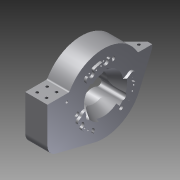
# Autodesk Inventor part: launcherhousing
Saved by Autodesk Inventor 2011 (Build 150239000, 239)
## iProperties
Created: 2011-01-27
Part Number: launcherhousing
Document SubType Name: Modeling
Designer: Casey
Density: 1 g/cm^3
Mass: 704.398 g
Surface Area: 699.987 cm^2
Volume: 704.398 cm^3
Author: Casey
Autodesk Inventor part; units mm, degrees
ref_plane "YZ Plane" through (0, 0, 0) normal (1, 0, 0) x (0, 1, 0)
ref_plane "XZ Plane" through (0, 0, 0) normal (0, 1, 0) x (-1, 0, 0)
ref_plane "XY Plane" through (0, 0, 0) normal (0, 0, 1) x (1, 0, 0)
sketch "Sketch1" plane through (0, 0, 0) normal (0, 0, 1) x (1, 0, 0)
  line L0 (2.0196, 25) -> (20, 35.381)
  line L1 (20, 35.381) -> (20, 70)
  line L2 (20, 70) -> (0, 70)
  line L3 (0, 0) -> (46.5621, 0) construction
  line L4 (0, 70) -> (0, 25)
  line L5 (0, 25) -> (2.0196, 25)
  line L6 (0, 25) -> (-20, 25)
  line L7 (-20, 25) -> (-20, 70)
  line L8 (-20, 70) -> (0, 70)
  dimension "d3" = 70
  dimension "d6" = 30
  dimension "d8" = 25
  dimension "d86" = 35.381
  dimension "d182" = 20
  dimension "d230" = 20
  constraints: 18 end point, 2 horizontal, 2 perpendicular, 2 vertical, 1 collinear, 1 parallel, 1 point on line, 1 other
  measures "d3" distance from line of L3.start L2
  measures "d6" angle of L5 L0
  measures "d8" distance from line of L3.start L5
  measures "d86" distance from line of L3 L0.end
  measures "d182" distance between parallel lines of L4 L1
  measures "d230" distance of L4.end L6.end
revolve "Revolution1" add sketch "Sketch1" angle 360 about axis through (0, 0, 0) along (1, 0, 0)
sketch "Sketch11" plane through (20, 0, 0) normal (1, 0, 0) x (0, 0, -1)
  circle A0 centre (0, 0) radius 35.381 projected
  line L0 (-35, -6) -> (0, -6)
  line L1 (0, -6) -> (0, 6)
  line L2 (0, 6) -> (-35, 6)
  arc A1 (-35, 6) -> (-35, -6) centre (-35, 0) ccw
  line L3 (-35, 0) -> (0, 0) construction
  dimension "d87" = 12
  dimension "d88" = 35
  constraints: 8 end point, 2 horizontal, 2 midpoint, 2 point on circle, 1 centre point, 1 parallel, 1 perpendicular, 1 point on line, 1 tangent
  measures "d87" diameter of A1
  measures "d88" distance of A0.centre L3.start
extrude "Extrusion10" cut sketch "Sketch11" against normal through all contours L2 L1 L0 A0 | A0 L0 A1 L2 picked at (-11.7746, -0.6695)
fillet "Fillet12" radius 20 2 edges at (-8.9902, 6, 24.2693) (-8.9902, -6, 24.2693)
pattern_circular "Circular Pattern6" count 3 over 360 about axis through (11.0098, 0, 0) along (1, 0, 0) of "Extrusion10", "Fillet12"
sketch "Sketch26" plane through (20, 0, 0) normal (1, 0, 0) x (0, 0, -1)
  arc A0 (12.2088, 33.2078) -> (12.5203, 33.6579) centre (-4.0786, 44.8148) ccw projected
  arc A1 (22.8885, 27.6719) -> (12.5203, 33.6579) centre (17.5, 30.3109) ccw projected
  arc A2 (22.8885, 27.6719) -> (22.6545, 27.177) centre (40.8501, 18.8752) ccw projected
  arc A3 (22.6545, -27.177) -> (22.6545, 27.177) centre (0, 0) ccw projected
  arc A4 (22.6545, -27.177) -> (22.8885, -27.6719) centre (40.8501, -18.8752) ccw projected
  arc A5 (12.5203, -33.6579) -> (22.8885, -27.6719) centre (17.5, -30.3109) ccw projected
  arc A6 (12.5203, -33.6579) -> (12.2088, -33.2078) centre (-4.0786, -44.8148) ccw projected
  arc A7 (-34.8632, -6.0308) -> (12.2088, -33.2078) centre (0, 0) ccw projected
  arc A8 (-34.8632, -6.0308) -> (-35.4088, -5.9861) centre (-36.7714, -25.9396) ccw projected
  arc A9 (-35.4088, 5.9861) -> (-35.4088, -5.9861) centre (-35, 0) ccw projected
  arc A10 (-35.4088, 5.9861) -> (-34.8632, 6.0308) centre (-36.7714, 25.9396) ccw projected
  arc A11 (12.2088, 33.2078) -> (-34.8632, 6.0308) centre (0, 0) ccw projected
  circle A12 centre (0, 0) radius 70 projected
  circle A13 centre (0, 0) radius 54.5
  dimension "d183" = 109
  constraints: 1 centre point, 1 coincident
  measures "d183" diameter of A13
extrude "Extrusion14" add sketch "Sketch26" along normal blind 4.5 contours A13
sketch "Sketch27" plane through (0, 0, 0) normal (0, 0, 1) x (1, 0, 0)
  line L0 (20, 35.381) -> (24.5, 37.9791)
  line L1 (24.5, 37.9791) -> (24.5, 35.381)
  line L2 (24.5, 35.381) -> (20, 35.381)
  line L3 (20, 35.381) -> (2.4267, 25.2351) projected
  line L4 (24.5, 54.5) -> (24.5, -54.5) projected
  line L5 (0, 0) -> (24.5, 0) construction
  constraints: 8 end point, 2 collinear, 1 midpoint, 1 perpendicular, 1 vertical
revolve "Revolution3" cut sketch "Sketch27" angle 360 about axis through (0, 0, 0) along (1, 0, 0)
sketch "Sketch28" plane through (24.5, 0, 0) normal (1, 0, 0) x (0, 0, -1)
  arc A0 (23.4822, -29.8495) -> (23.4822, 29.8495) centre (0, 0) ccw projected
  arc A1 (14.1093, 35.261) -> (-37.5916, 5.4114) centre (0, 0) ccw projected
  circle A2 centre (0, 0) radius 54.5 construction
  arc A3 (-51.2132, 18.6401) -> (-43.046, 12.1486) centre (-46.0449, 16.759) ccw
  circle A4 centre (-46.0449, 16.759) radius 4 construction
  line L0 (0, 0) -> (-46.0449, 16.759) construction
  line L1 (0, 0) -> (-54.5, 0) construction
  arc A5 (-35.6887, 12.9896) -> (-43.046, 12.1486) centre (-38.5247, 5.1978) ccw
  line L2 (0, 0) -> (-27.25, 47.1984) construction
  line L3 (0, 0) -> (-41.7494, 35.0319) construction
  line L4 (0, 0) -> (-9.4638, 53.672) construction
  arc A6 (-6.595, 37.4021) -> (-18.0868, 51.4113) centre (-46.0449, 16.759) ccw
  arc A7 (-18.0868, 51.4113) -> (-51.2132, 18.6401) centre (0, 0) ccw
  line L5 (-35.6887, 12.9896) -> (0, 0)
  line L6 (0, 0) -> (-1.9138, 10.8535)
  arc A8 (-1.9138, 10.8535) -> (-6.595, 37.4021) centre (-46.0449, 16.759) ccw
  dimension "d187" = 11
  dimension "d188" = 8
  dimension "d190" = 20
  dimension "d191" = 60
  dimension "d192" = 20
  constraints: 18 point on circle, 14 end point, 6 centre point, 5 point on line, 4 tangent, 3 coincident, 2 collinear, 2 concentric, 1 horizontal, 1 other
  measures "d187" diameter of A3
  measures "d188" diameter of A4
  measures "d190" angle of L1 L0
  measures "d191" angle of L1 L2
  measures "d192" angle of L2 L3
extrude "Extrusion15" cut sketch "Sketch28" against normal up to surface (4.5 mm away)
fillet "Fillet13" radius 6 2 edges at (22.25, 18.6401, 51.2132) (22.25, 51.4113, 18.0868)
sketch "Sketch30" plane through (24.5, 0, 0) normal (1, 0, 0) x (0, 0, -1)
  arc A0 (14.1093, 35.261) -> (-6.595, 37.4021) centre (0, 0) ccw projected
  arc A1 (-54.1534, 6.1367) -> (-7.1884, 54.0239) centre (0, 0) ccw projected
  circle A2 centre (-51, 0) radius 5
  circle A3 centre (0, 51) radius 5
  line L0 (-51, 0) -> (0, 0) construction
  line L1 (0, 0) -> (0, 51) construction
  dimension "d199" = 51
  dimension "d200" = 10
  dimension "d201" = 90
  constraints: 4 end point, 2 centre point, 1 equal radius, 1 horizontal, 1 perpendicular
  measures "d199" distance of A0.centre L0.start
  measures "d200" diameter of A2
  measures "d201" angle of L0 L1
extrude "Extrusion17" cut sketch "Sketch30" against normal up to surface (4.5 mm away)
sketch "Sketch29" plane through (20, 0, 0) normal (1, 0, 0) x (0, 0, -1)
  arc A0 (-5.4125, 34.9645) -> (-11.1054, 44.3572) centre (-46.0449, 16.759) ccw projected
  circle A1 centre (-46.0449, 16.759) radius 4
  arc A2 (-3.6891, 54.375) -> (3.6891, 54.375) centre (0, 51) ccw projected
  arc A3 (-54.375, -3.6891) -> (-54.375, 3.6891) centre (-51, 0) ccw projected
  circle A4 centre (-51, 0) radius 1.5
  circle A5 centre (0, 51) radius 1.5
  dimension "d196" = 8
  dimension "d205" = 3
  constraints: 3 centre point, 3 coincident, 1 equal radius
  measures "d196" diameter of A1
  measures "d205" diameter of A4
extrude "Extrusion16" cut sketch "Sketch29" against normal blind 4
fillet "Fillet14" radius 2 4 edges at (22.25, 54.375, 3.6891) (22.25, 54.375, -3.6891) (22.25, -3.6891, 54.375) (22.25, 3.6891, 54.375)
sketch "Sketch32" plane through (24.5, 0, 0) normal (1, 0, 0) x (0, 0, -1)
  arc A0 (-4.9443, 51.744) -> (4.9443, 51.744) centre (0, 51) ccw projected
  arc A1 (-35.6887, 12.9896) -> (-37.5916, 5.4114) centre (0, 0) ccw projected
  circle A2 centre (8.769, 49.7316) radius 1.5
  line L0 (0, 0) -> (8.769, 49.7316) construction
  line L1 (0, 0) -> (17.2716, 47.4533) construction
  circle A3 centre (17.2716, 47.4533) radius 1.5
  line L2 (0, 0) -> (0, 51) construction
  dimension "d212" = 10
  dimension "d213" = 3
  dimension "d214" = 10
  constraints: 6 end point, 2 centre point, 1 coincident, 1 equal length, 1 equal radius, 1 vertical
  measures "d212" angle of L0 L1
  measures "d213" diameter of A2
  measures "d214" angle of L2 L0
extrude "Extrusion18" cut sketch "Sketch32" against normal blind 6
pattern_circular "Circular Pattern7" count 3 over 360 about axis through (11.0098, 0, 0) along (1, 0, 0) of "Fillet14", "Extrusion16", "Extrusion17", "Fillet13", "Extrusion15", "Extrusion18"
sketch "Sketch37" plane through (20, 0, 0) normal (1, 0, 0) x (0, 0, -1)
  circle A0 centre (0, 0) radius 70 projected
  line L0 (0, 0) -> (-70, 0)
  line L1 (-33, 127.5928) -> (-33, -153.3299)
  line L2 (-33, 87.6343) -> (-27, 87.6343)
  line L3 (-27, 87.6343) -> (27.4797, 64.3806)
  line L4 (-33, -101.0161) -> (46.9095, -101.0161)
  line L5 (46.9095, -101.0161) -> (67.9117, -16.9705)
  line L6 (0, 70) -> (-67.7664, 70) construction
  arc A1 (-33, -61.7333) -> (67.9117, -16.9705) centre (0, 0) ccw
  arc A2 (27.4797, 64.3806) -> (-33, 61.7333) centre (0, 0) ccw
  line L7 (-33, 61.7333) -> (-33, 87.6343)
  line L8 (-33, -61.7333) -> (-33, -101.0161)
  dimension "d224" = 37
  dimension "d249" = 188.6504
  dimension "d250" = 101.0161
  dimension "d251" = 79.9095
  dimension "d252" = 6
  constraints: 18 end point, 10 point on circle, 4 point on line, 4 tangent, 3 perpendicular, 2 centre point, 2 collinear, 2 concentric, 1 horizontal, 1 parallel
  measures "d224" distance from line of L1 L0.end
  measures "d249" distance between parallel lines of L4 L2
  measures "d250" distance between parallel lines of L4 L0
  measures "d251" distance of L4.start L4.end
  measures "d252" distance of L2.start L2.end
extrude "Extrusion20" add sketch "Sketch37" against normal up to surface (40 mm away) contours A0 L1 L2 L3 | L5 L4 L1 A0
fillet "Fillet15" radius 3 2 edges at (0, -61.7333, 33) (0, 61.7333, 33)
fillet "Fillet16" radius 20 2 edges at (0, -101.0161, -46.9095) (0, 87.6343, 27)
sketch "Sketch39" plane through (-20, 87.6343, 33) normal (0, 0, 1) x (1, 0, 0)
  line L0 (40, 0) -> (0, 0) projected
  line L1 (0, -151.1402) -> (40, -151.1402) projected
  line L2 (0, -151.1402) -> (0, -188.6504) projected
  line L3 (40, -188.6504) -> (0, -188.6504) projected
  line L4 (40, -151.1402) -> (40, -188.6504) projected
  circle A0 centre (28.5, -12.6343) radius 3
  circle A1 centre (11.5, -12.6343) radius 3
  line L5 (20, 0) -> (20, -208.8671)
  line L6 (28.5, -12.6343) -> (28.5, -208.8671)
  line L7 (11.5, -12.6343) -> (11.5, -208.5633)
  line L8 (11.5, -12.6343) -> (28.5, -12.6343)
  circle A2 centre (28.5, -160.6343) radius 3
  circle A3 centre (11.5, -160.6343) radius 3
  circle A4 centre (28.5, -178.6343) radius 3
  circle A5 centre (11.5, -178.6343) radius 3
  line L9 (11.5, -160.6343) -> (28.5, -160.6343)
  line L10 (11.5, -178.6343) -> (28.5, -178.6343)
  line L11 (0, 0) -> (0, -24.1284) projected
  line L12 (20, -87.6343) -> (-34.952, -87.6343)
  dimension "d231" = 6
  dimension "d232" = 6
  dimension "d233" = 6
  dimension "d234" = 6
  dimension "d235" = 6
  dimension "d236" = 6
  dimension "d253" = 148
  dimension "d254" = 18
  dimension "d255" = 75
  dimension "d256" = 8.5
  constraints: 14 end point, 6 centre point, 4 perpendicular, 4 point on line, 3 parallel, 1 midpoint, 1 other
  measures "d231" diameter of A0
  measures "d232" diameter of A1
  measures "d233" diameter of A2
  measures "d234" diameter of A3
  measures "d235" diameter of A4
  measures "d236" diameter of A5
  measures "d253" distance between parallel lines of L8 L9
  measures "d254" distance between parallel lines of L9 L10
  measures "d255" distance between parallel lines of L8 L12
  measures "d256" distance between parallel lines of L5 L7
hole "Hole5" at (8.5, 75, 33) at (-8.5, 75, 33) at (8.5, -73, 33) at (8.5, -91, 33) at (-8.5, -91, 33) at (-8.5, -73, 33) direction (0, 0, -1) diameter 4.917 depth 8 tip angle 118 thread size "M6x1" class "6H" standard "ANSI Metric M Profile"
sketch "Sketch41" plane through (20, -101.0161, 33) normal (1, 0, 0) x (0, 0, -1)
  line L0 (0, 0) -> (64.2923, 0) projected
  arc A0 (100.9117, 84.0455) -> (60.4797, 165.3967) centre (33, 101.0161) ccw projected
  line L1 (33, 101.0161) -> (13.4499, 35.0161)
  circle A1 centre (13.4499, 35.0161) radius 2.3812
  line L2 (33, 101.0161) -> (33, 18.7551) construction
  dimension "d244" = 4.7625
  dimension "d245" = 16.5
  dimension "d248" = 66
  constraints: 4 end point, 1 centre point, 1 coincident, 1 perpendicular
  measures "d244" diameter of A1
  measures "d245" angle of L2 L1
  measures "d248" vertical distance of L1.start L1.end
extrude "Extrusion21" cut sketch "Sketch41" against normal blind 51.5
sketch "Sketch42" plane through (-20, 87.6343, 33) normal (0, 0, 1) x (1, 0, 0)
  circle A0 centre (11.5, -12.6343) radius 2.4585 projected
  line L0 (40, 0) -> (0, 0) projected
  line L1 (0, 0) -> (0, -24.1284) projected
  line L2 (32.2214, 0) -> (0, -31.2634)
  line L3 (0, -31.2634) -> (0, 0)
  line L4 (32.2214, 0) -> (0, 0)
  point P0 (20, -87.6343)
  constraints: 6 end point, 2 collinear, 1 point on line
extrude "Extrusion22" cut sketch "Sketch42" against normal through all contours A0 | L2 L3 L1 L0
sketch "Sketch43" plane through (-20, 87.6343, 33) normal (0, 0, -1) x (-1, 0, 0)
  line L0 (-7.3536, -24.1284) -> (0, -24.1284) projected
  line L1 (0, -31.2634) -> (-7.3536, -24.1284) projected
  line L2 (0, -24.1284) -> (0, -31.2634) projected
  point P0 (-20, -87.6343)
extrude "Extrusion23" cut sketch "Sketch43" against normal through all
body "Solid1"
